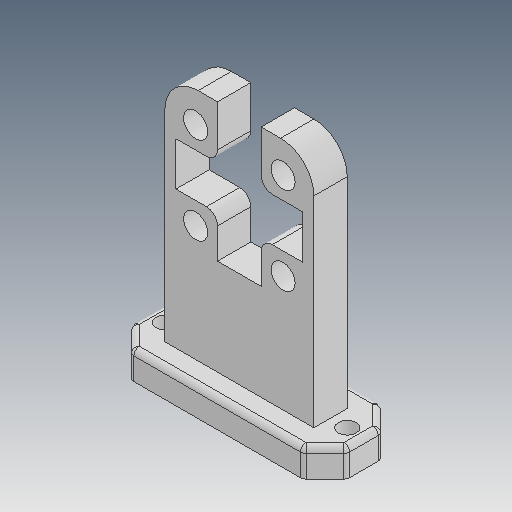
# Autodesk Inventor part: as5600mount_2
Saved by Autodesk Inventor 2025.2 (Build 292293000, 293)
## iProperties
Created: 2025-02-16
Part Number: as5600mount_2
Material: Generic
Document SubType Name: Modeling
Designer: turbo
Density: 1 g/cm^3
Appearance: Default
Author: turbo
Autodesk Inventor part; units mm, degrees
ref_plane "YZ Plane" through (0, 0, 0) normal (1, 0, 0) x (0, 1, 0)
ref_plane "XZ Plane" through (0, 0, 0) normal (0, 1, 0) x (-1, 0, 0)
ref_plane "XY Plane" through (0, 0, 0) normal (0, 0, 1) x (1, 0, 0)
sketch "Sketch1" plane through (0, 0, 0) normal (0, 0, 1) x (1, 0, 0)
  line L0 (0, 0) -> (26.86, 0)
  line L1 (26.86, 0) -> (26.86, 47.18)
  line L2 (26.86, 47.18) -> (0, 47.18)
  line L3 (0, 47.18) -> (0, 0)
  line L4 (2, 38.68) -> (8.5, 38.68)
  line L5 (8.5, 38.68) -> (8.5, 45.18)
  line L6 (8.5, 45.18) -> (18.36, 45.18)
  line L7 (18.36, 45.18) -> (18.36, 38.68)
  line L8 (18.36, 38.68) -> (24.86, 38.68)
  line L9 (24.86, 38.68) -> (24.86, 28.82)
  line L10 (24.86, 28.82) -> (18.36, 28.82)
  line L11 (18.36, 28.82) -> (18.36, 22.32)
  line L12 (18.36, 22.32) -> (8.5, 22.32)
  line L13 (8.5, 22.32) -> (8.5, 28.82)
  line L14 (2, 28.82) -> (2, 38.68)
  line L15 (2, 28.82) -> (8.5, 28.82)
  line L16 (2, 33.75) -> (24.86, 33.75) construction
  line L17 (13.43, 47.18) -> (13.43, 0) construction
  circle A0 centre (5.556, 41.624) radius 2.175
  circle A1 centre (5.556, 25.876) radius 2.175
  circle A2 centre (21.304, 25.876) radius 2.175
  circle A3 centre (21.304, 41.624) radius 2.175
  line L18 (8.5, 45.18) -> (8.5, 47.18)
  line L19 (18.36, 45.18) -> (18.36, 47.18)
  line L20 (5.556, 41.624) -> (21.304, 41.624)
  line L21 (21.304, 41.624) -> (21.304, 25.876)
  line L22 (21.304, 25.876) -> (5.556, 25.876)
  line L23 (5.556, 25.876) -> (5.556, 41.624)
  line L24 (26.86, 47.18) -> (17.36, 47.18)
  line L25 (17.36, 47.18) -> (17.36, 37.68)
  line L26 (17.36, 37.68) -> (26.86, 37.68)
  line L27 (26.86, 37.68) -> (26.86, 47.18)
  line L28 (0, 47.18) -> (9.5, 47.18)
  line L29 (9.5, 47.18) -> (9.5, 37.68)
  line L30 (9.5, 37.68) -> (0, 37.68)
  line L31 (0, 37.68) -> (0, 47.18)
  line L32 (0, 20.8011) -> (9.5, 20.8011)
  line L33 (9.5, 20.8011) -> (9.5, 29.82)
  line L34 (9.5, 29.82) -> (0, 29.82)
  line L35 (0, 29.82) -> (0, 20.8011)
  line L36 (26.86, 20.8011) -> (17.36, 20.8011)
  line L37 (17.36, 20.8011) -> (17.36, 29.82)
  line L38 (17.36, 29.82) -> (26.86, 29.82)
  line L39 (26.86, 29.82) -> (26.86, 20.8011)
  point P0 (13.43, 33.75)
  point P1 (5.25, 38.68)
  point P2 (9.5, 22.32)
  point P3 (2, 29.82)
  point P4 (5.556, 28.82)
  point P5 (5.556, 28.051)
  point P6 (7.731, 25.876)
  point P7 (8.5, 25.876)
  point P8 (17.36, 22.32)
  point P9 (18.36, 25.876)
  point P10 (19.129, 25.876)
  point P11 (21.304, 28.051)
  point P12 (21.304, 28.82)
  point P13 (24.86, 29.82)
  point P14 (24.86, 37.68)
  point P15 (21.304, 38.68)
  point P16 (21.304, 39.449)
  point P17 (19.129, 41.624)
  point P18 (18.36, 41.624)
  point P19 (8.5, 41.624)
  point P20 (7.731, 41.624)
  point P21 (5.556, 39.449)
  point P22 (5.556, 38.68)
  point P23 (2, 37.68)
  dimension "d0" = 47.18
  dimension "d1" = 26.86
  dimension "d2" = 6.5
  dimension "d3" = 22.86
  dimension "d4" = 2
  dimension "d5" = 4.35
  dimension "d6" = 2.944
  dimension "d7" = 2.944
  dimension "d19" = 15.748
  dimension "d20" = 15.748
  dimension "d21" = 1
  dimension "d22" = 1
  dimension "d23" = 1
  dimension "d24" = 1
  constraints: 80 end point, 15 parallel, 14 perpendicular, 12 point on line, 8 equal length, 8 horizontal, 6 midpoint, 4 centre point, 3 equal radius, 2 horizontal alignment, 2 vertical alignment, 2 other
  measures "d0" distance of L0.end L1.end
  measures "d1" distance of L0.start L0.end
  measures "d2" distance of L7.end L8.end
  measures "d3" distance between parallel lines of L6 L12
  measures "d4" distance between parallel lines of L2 L6
  measures "d5" diameter of A0
  measures "d6" distance from line of L5 L20.start
  measures "d7" vertical distance of L20.start point (5.25, 38.68)
  measures "d19" distance of L22.end L20.start
  measures "d20" distance of L21.end L22.end
  measures "d21" distance between parallel lines of L5 L29
  measures "d22" distance between parallel lines of L4 L30
  measures "d23" distance between parallel lines of L10 L38
  measures "d24" distance between parallel lines of L11 L37
extrude "Extrusion1" add sketch "Sketch1" along normal blind 6 contours L3 L32 L33 L12 L37 L36 L1 L0 | L3 L34 L14 L15 L23 A1 L22 L13 L12 L33 L32 | L36 L37 L12 L11 L22 A2 L21 L10 L9 L38 L1 | L3 L30 L14 L34 | L38 L9 L26 L1 | L3 L2 L18 L5 L20 A0 L23 L4 L14 L30 | L26 L9 L8 L21 A3 L20 L7 L19 L2 L1 | L15 L13 L22 A1 L23 | L21 A2 L22 L11 L10 | L23 A0 L20 L5 L4 | L8 L7 L20 A3 L21
fillet "Fillet1" radius 2 4 edges at (8.5, 28.82, 3) (18.36, 28.82, 3) (8.5, 38.68, 3) (18.36, 38.68, 3)
fillet "Fillet2" radius 6 2 edges at (0, 47.18, 3) (26.86, 47.18, 3)
sketch "Sketch2" plane through (0, 0, 6) normal (0, 0, 1) x (1, 0, 0)
  line L0 (8.5, 45.18) -> (18.36, 45.18)
  line L1 (24.86, 38.68) -> (24.86, 28.82) projected
  line L2 (18.36, 22.32) -> (8.5, 22.32) projected
  line L3 (2, 28.82) -> (2, 38.68) projected
  circle A0 centre (13.43, 33.75) radius 11.43
  point P0 (0, 0)
  constraints: 3 tangent, 2 end point, 1 centre point
sketch "Sketch3" plane through (0, 0, 0) normal (0, -1, 0) x (1, 0, 0)
  line L0 (0, 0) -> (26.86, 0) construction
  line L1 (26.86, 0) -> (26.86, 6) construction
  line L2 (0, 6) -> (26.86, 6) construction
  line L3 (0, 0) -> (0, 6) construction
  line L4 (-6, 6) -> (32.86, 6) construction
  line L5 (32.86, 6) -> (32.86, 0)
  line L6 (32.86, 0) -> (-6, 0) construction
  line L7 (-6, 0) -> (-6, 6)
  line L8 (0, 6) -> (26.86, 6) projected
  line L9 (0, 0) -> (26.86, 0) projected
  line L10 (13.43, 6) -> (13.43, 0) construction
  line L11 (13.43, 6) -> (13.43, 0) construction
  circle A0 centre (29.86, 3) radius 1.625
  line L12 (26.86, 6) -> (32.86, 0) construction
  circle A1 centre (-3, 3) radius 1.625
  line L13 (-6, 0) -> (-2, -4)
  line L14 (-2, -4) -> (28.86, -4)
  line L15 (28.86, -4) -> (32.86, 0)
  line L16 (-6, 6) -> (-2, 10)
  line L17 (-2, 10) -> (28.86, 10)
  line L18 (28.86, 10) -> (32.86, 6)
  line L19 (0, 0) -> (0, 6) projected
  line L20 (0, 6) -> (0, 0)
  line L21 (26.86, 0) -> (26.86, 6) projected
  line L22 (26.86, 6) -> (26.86, 0)
  point P0 (13.43, 3)
  dimension "d12" = 6
  dimension "d13" = 3.25
  dimension "d14" = 6
  dimension "d15" = 4
  constraints: 30 end point, 7 midpoint, 4 equal length, 3 parallel, 2 centre point, 2 collinear, 2 horizontal, 2 perpendicular, 2 vertical, 1 coincident, 1 symmetric about line, 1 other
  measures "d12" distance between parallel lines of L5 L1
  measures "d13" diameter of A0
  measures "d14" distance between parallel lines of L3 L7
  measures "d15" distance between parallel lines of L17 L4
extrude "Extrusion2" add sketch "Sketch3" against normal blind 5
fillet "Fillet3" radius 1 16 edges at (13.43, 5, 10) (-6, 5, 3) (-4, 5, 8) (-4, 5, -2) (13.43, 5, -4) (30.86, 5, 8) (32.86, 5, 3) (30.86, 5, -2) (-6, 2.5, 0) (-6, 2.5, 6) (28.86, 2.5, 10) (-2, 2.5, 10) (32.86, 2.5, 6) (32.86, 2.5, 0) (28.86, 2.5, -4) (-2, 2.5, -4)
extrude "Extrusion3" add sketch "Sketch1" along normal blind 6 contours L34 L23 L15 L14 | L12 L13 L22 L33 | L9 L10 L21 L38 | L37 L22 L11 L12 | L14 L4 L23 L30 | L34 L33 L22 L13 L15 L23 | L26 L21 L8 L9 | L21 L10 L11 L22 L37 L38 | L2 L29 L6 L18 | L23 L4 L5 L20 L29 L30 | L15 L13 L22 A1 L23 | L19 L6 L25 L2 | L26 L25 L20 L7 L8 L21 | L21 A2 L22 L11 L10 | L6 L29 L20 L5 | L23 A0 L20 L5 L4 | L7 L20 L25 L6 | L8 L7 L20 A3 L21
fillet "Fillet4" radius 2 4 edges at (9.5, 37.68, 3) (17.36, 37.68, 3) (9.5, 29.82, 3) (17.36, 29.82, 3)
body "Solid1"
